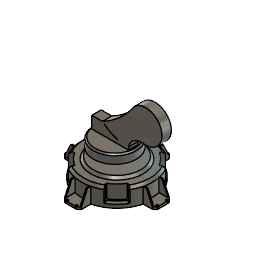
Robotic_Arm (Autodesk Fusion 360 design; units mm, degrees)
part number: 2026-03-02-22-55-42-666
part number: 2026-03-02-23-27-00-819
part number: 2026-03-03-10-06-11-483
part number: 2026-03-03-11-15-49-242
Autodesk Fusion 360 part; units mm, degrees
note: some values were not read from the file. Chosen so that the rebuilt part matches the saved one: which face or edge a step refers to; that a step has no effect. Set by a fixed rule: which sketch regions a step uses.
sketch "Sketch1" plane through (0, 0, 0) normal (0, 1, 0) x (1, 0, 0) in component "Base of thr Arm"
  circle A0 centre (0, 0) radius 150
  dimension "d1" = 300
  constraint coincident A0.centre origin
  measures "d1" diameter of A0
extrude "Extrude1" add sketch "Sketch1" along normal blind 75 makes body 1 in component "Base of thr Arm"
chamfer "Chamfer1" distance 10 angle 45 1 edges at (-139.8491, 75, 54.2423) on bodies 1 in component "Base of thr Arm"
sketch "Sketch1 (2)" plane through (0, 0, 0) normal (0, 1, 0) x (1, 0, 0)
  line L0 (-195.7386, 0) -> (-195.7386, 35.5)
  line L1 (-195.7386, 0) -> (-195.7386, -35.5)
  line L2 (-195.7386, 35.5) -> (-145.7386, 35.5)
  line L3 (-195.7386, -35.5) -> (-145.7386, -35.5)
  circle A0 centre (0, 0) radius 150
  dimension "d23" = 35.5
  dimension "d24" = 35.5
  dimension "d25" = 50
  dimension "d26" = 50
  constraint vertical L0
  constraint vertical L1
  constraint perpendicular L0 L2
  constraint perpendicular L1 L3
  constraint coincident L2.end A0
  constraint coincident L3.end A0
  measures "d23" distance of L0.start L0.end
  measures "d24" distance of L0.start L1.end
  measures "d25" distance of L0.end L2.end
  measures "d26" distance of L1.end L3.end
extrude "Extrude1'" add sketch "Sketch1 (2)" along normal blind 10 separate body contours L0 L1 L2 L3 A0 makes body 2 in component "Scerw holder"
sketch "Sketch1 (3)" plane through (0, 0, 35.5) normal (0, 0, 1) x (1, 0, 0) in component "Scerw holder"
  line L0 (-195.7386, 0) -> (-145.7386, 0)
  line L1 (-145.7386, 0) -> (-145.7386, 10)
  line L2 (-145.7386, 10) -> (-195.7386, 10)
  line L3 (-195.7386, 10) -> (-195.7386, 0)
  line L4 (-145.7386, 10) -> (-145.7386, 65)
  line L5 (-145.7386, 65) -> (-160, 65)
  line L6 (-160, 65) -> (-185, 10)
  line L7 (-145.7386, 10) -> (-185, 10)
  constraint coincident L1.end L2.start
  constraint perpendicular L2 L4
  constraint perpendicular L4 L5
  constraint coincident L2 L6.end
extrude "Extrude3" add sketch "Sketch1 (3)" against normal blind 5 contours L2 L4 L5 L6 L7 bodies 2 in component "Scerw holder"
chamfer "Chamfer2" distance 10.5 angle 45 2 edges at (-195.7386, 5, -35.5) (-195.7386, 5, 35.5) on bodies 2 in component "Scerw holder"
sketch "Sketch2" plane through (0, 10, 0) normal (0, 1, 0) x (-1, 0, 0) in component "Scerw holder"
  line L0 (195.7386, 25) -> (185.2386, 35.5)
  line L1 (185.2386, 35.5) -> (185, 35.5)
  line L2 (185, 35.5) -> (185, 30.5)
  line L3 (185, 30.5) -> (146.8664, 30.5)
  arc A0 (145.7386, -35.5) -> (146.8664, 30.5) centre (0, 0) ccw
  line L4 (145.7386, -35.5) -> (185.2386, -35.5)
  line L5 (185.2386, -35.5) -> (195.7386, -25)
  line L6 (195.7386, -25) -> (195.7386, 25)
  line L7 (194, 22.3094) -> (190, 24.6188)
  line L8 (190, 24.6188) -> (186, 22.3094)
  line L9 (186, 22.3094) -> (186, 17.6906)
  line L10 (186, 17.6906) -> (190, 15.3812)
  line L11 (190, 15.3812) -> (194, 17.6906)
  line L12 (194, 17.6906) -> (194, 22.3094)
  point P0 (190, 20)
extrude "Extrude4" cut sketch "Sketch2" against normal blind 10 contours L7 L8 L9 L10 L11 L12 bodies 2 in component "Scerw holder"
mirror "Mirror2" about plane through (0, 0, 0) normal (0, 0, 1) of "Extrude3", "Extrude4" in component "Scerw holder"
pattern_circular "C-Pattern1" count 4 over 360 about axis through (0, 1.75, 0) along (0, 1, 0) of bodies 2 makes body 3 at (0, 0, 174) makes body 4 at (174, 0, 0) makes body 5 at (0, 0, -174) in component "Scerw holder"
sketch "Sketch5" plane through (0, 75, 0) normal (0, 1, 0) x (-1, 0, 0) in component "Base of thr Arm"
  circle A0 centre (0, 0) radius 140
  line L0 (0, 0) -> (170, 0)
  line L1 (0, 0) -> (0, 150)
  line L2 (0, 0) -> (174.0838, 100.5073)
  line L3 (0, 0) -> (105.4587, 182.6598)
  circle A1 centre (0, 0) radius 130
  circle A2 centre (0, 0) radius 150
  dimension "d47" = 30
  dimension "d48" = 30
  dimension "d49" = 260
  dimension "d50" = 300
  constraint coincident A0.centre L0.start
  constraint horizontal L0
  constraint perpendicular L0 L1
  measures "d47" angle of L0 L2
  measures "d48" angle of L1 L3
  measures "d49" diameter of A1
  measures "d50" diameter of A2
extrude "Extrude6" cut sketch "Sketch5" against normal blind 60 contours A0 L2 L3 A1 | A0 L2 L3 A2 bodies 1 in component "Base of thr Arm"
fillet "Fillet1" radius 3 5 edges at (-112.5833, 45, 65) (-65, 45, 112.5833) (-91.9239, 15, 91.9239) (-121.2436, 15, 70) (-70, 15, 121.2436) on bodies 1 in component "Base of thr Arm"
pattern_circular "C-Pattern1'" count 4 over 360 about axis through (0, 1.75, 0) along (0, 1, 0) of 11 faces at (-105.3564, 37, 76.1579) (-112.4433, 37, 66.3355) (-112.3586, 17.6084, 66.4028) (-123.6174, 15.0142, 74.498) (-120.0379, 15, 79.7213) (-76.2075, 17.2927, 105.4249) (-66.1107, 17.6084, 113.5001) (-66.2488, 37, 114.641) (-69.3221, 52.6667, 120.0693) (-73.7477, 15.2347, 124.0613) (-120.0693, 52.6667, 69.3221) on bodies 1 in component "Base of thr Arm"
sketch "Sketch6" plane through (0, 75, 0) normal (0, 1, 0) x (-1, 0, 0) in component "Base of thr Arm"
  line L0 (115.1521, -66.4831) -> (121.2436, -70)
  arc A0 (121.2436, -70) -> (121.2436, 70) centre (0, 0) ccw
  line L1 (121.2436, 70) -> (115.1521, 66.4831)
  arc A1 (111.0885, 67.5229) -> (115.1521, 66.4831) centre (113.6521, 69.0812) ccw
  arc A2 (111.0885, 67.5229) -> (67.5229, 111.0885) centre (0, 0) ccw
  arc A3 (66.4831, 115.1521) -> (67.5229, 111.0885) centre (69.0812, 113.6521) ccw
  line L2 (66.4831, 115.1521) -> (70, 121.2436)
  arc A4 (70, 121.2436) -> (-70, 121.2436) centre (0, 0) ccw
  line L3 (-70, 121.2436) -> (-66.4831, 115.1521)
  arc A5 (-67.5229, 111.0885) -> (-66.4831, 115.1521) centre (-69.0812, 113.6521) ccw
  arc A6 (-67.5229, 111.0885) -> (-111.0885, 67.5229) centre (0, 0) ccw
  arc A7 (-115.1521, 66.4831) -> (-111.0885, 67.5229) centre (-113.6521, 69.0812) ccw
  line L4 (-115.1521, 66.4831) -> (-121.2436, 70)
  arc A8 (-121.2436, 70) -> (-121.2436, -70) centre (0, 0) ccw
  line L5 (-121.2436, -70) -> (-115.1521, -66.4831)
  arc A9 (-111.0885, -67.5229) -> (-115.1521, -66.4831) centre (-113.6521, -69.0812) ccw
  arc A10 (-111.0885, -67.5229) -> (-67.5229, -111.0885) centre (0, 0) ccw
  arc A11 (-66.4831, -115.1521) -> (-67.5229, -111.0885) centre (-69.0812, -113.6521) ccw
  line L6 (-66.4831, -115.1521) -> (-70, -121.2436)
  arc A12 (-70, -121.2436) -> (70, -121.2436) centre (0, 0) ccw
  line L7 (70, -121.2436) -> (66.4831, -115.1521)
  arc A13 (67.5229, -111.0885) -> (66.4831, -115.1521) centre (69.0812, -113.6521) ccw
  arc A14 (67.5229, -111.0885) -> (111.0885, -67.5229) centre (0, 0) ccw
  arc A15 (115.1521, -66.4831) -> (111.0885, -67.5229) centre (113.6521, -69.0812) ccw
  circle A16 centre (0, 0) radius 110
  dimension "d57" = 220
  constraint concentric A0 A16
  measures "d57" diameter of A16
extrude "Extrude7" add sketch "Sketch6" along normal blind 10 draft -45 contours A16 bodies 1 in component "Base of thr Arm"
sketch "Sketch7" plane through (0, 85, 0) normal (0, 1, 0) x (-1, 0, 0) in component "Base of thr Arm"
  circle A0 centre (0, 0) radius 100
  circle A1 centre (0, 0) radius 15
  dimension "d60" = 30
  constraint coincident A0.centre A1.centre
  measures "d60" diameter of A1
extrude "Extrude8" add sketch "Sketch7" along normal blind 20 contours A1 bodies 1 in component "Base of thr Arm"
sketch "Sketch1 (4)" plane through (0, 0, 0) normal (0, 1, 0) x (1, 0, 0) in component "Arm Jaw"
  circle A0 centre (0, 0) radius 90
  dimension "d63" = 180
  constraint coincident A0.centre origin
  measures "d63" diameter of A0
extrude "Extrude1''" add sketch "Sketch1 (4)" along normal blind 37 separate body makes body 6 in component "Arm Jaw"
chamfer "Chamfer1'" distance 6 angle 45 1 edges at (-83.9095, 37, 32.5454) on bodies 6 in component "Arm Jaw"
sketch "Sketch2 (2)" plane through (0, 37, 0) normal (0, 1, 0) x (-1, 0, 0) in component "Arm Jaw"
  circle A0 centre (0, 0) radius 84
  line L0 (77.5, 20) -> (-77.5, 20)
  line L1 (-77.5, 20) -> (-77.5, -20)
  line L2 (-77.5, -20) -> (77.5, -20)
  line L3 (77.5, -20) -> (77.5, 20)
  line L4 (77.5, 20) -> (-77.5, -20) construction
  line L5 (-77.5, 20) -> (77.5, -20) construction
  dimension "d67" = 155
  dimension "d68" = 40
  constraint horizontal L0
  constraint perpendicular L0 L1
  constraint parallel L0 L2
  constraint parallel L1 L3
  constraint coincident L4 A0.centre
  constraint coincident L5 A0.centre
  constraint coincident A0.centre origin
  measures "d67" distance of L1.end L2.end
  measures "d68" distance of L0.end L1.end
extrude "Extrude2" add sketch "Sketch2 (2)" along normal blind 50 contours L0 L1 L2 L3 bodies 6 in component "Arm Jaw"
sketch "Sketch3" plane through (0, 0, -20) normal (0, 0, -1) x (-1, 0, 0) in component "Arm Jaw"
  line L0 (-77.5, 37) -> (77.5, 37)
  line L1 (77.5, 37) -> (77.5, 87)
  line L2 (77.5, 87) -> (-77.5, 87)
  line L3 (-77.5, 87) -> (-77.5, 37)
  line L4 (-77.5, 87) -> (5.9265, 87)
  line L5 (-77.5, 87) -> (32.5, 87)
  line L6 (-77.5, 87) -> (-77.5, 48)
  arc A0 (-77.5, 48) -> (32.5, 87) centre (-70.2732, 202.2449) ccw
  dimension "d71" = 110
  dimension "d72" = 39
  constraint coincident L2.end L3.start
  constraint coincident L2 L4.end
  constraint perpendicular L3 L5
  constraint perpendicular L5 L6
  measures "d71" distance of L2.end L5.end
  measures "d72" distance of L2.end L6.end
extrude "Extrude3'" cut sketch "Sketch3" against normal blind 80 contours L2 L3 L4 L5 L6 A0 bodies 6 in component "Arm Jaw"
sketch "Sketch4" plane through (0, 0, 0) normal (0, 0, 1) x (1, 0, 0) in component "Arm Jaw"
  line L0 (0, 0) -> (150, 0)
  line L1 (150, 0) -> (150, 160)
  circle A0 centre (150, 160) radius 68.5
  arc A1 (139.9423, 92.2424) -> (77.3691, 47.5292) centre (131.8134, 37.4782) ccw
  arc A2 (-32.5378, 86.9467) -> (99.6249, 206.4177) centre (-205.8032, 411.4553) ccw
  arc A3 (-32.5378, 86.9467) -> (77.3691, 47.5292) centre (72.3379, 206.4349) ccw
  dimension "d75" = 160
  dimension "d76" = 137
  constraint coincident L0.start origin
  constraint horizontal L0
  constraint perpendicular L0 L1
  constraint coincident L1.end A0.centre
  constraint tangent A0 A1
  constraint coincident A0 A1.start
  constraint coincident A0 A2.end
  constraint tangent A0 A3
  measures "d75" distance of L0.end L1.end
  measures "d76" diameter of A0
extrude "Extrude4'" add sketch "Sketch4" along normal mid plane 40 contours A0 A2 | A0 A1 A2 A3 picked at (167.4331, 144.9511) bodies 6 in component "Arm Jaw"
sketch "Sketch2 (3)" plane through (0, 0, 35.5) normal (0, 0, 1) x (1, 0, 0)
  line L0 (-185.2386, 0) -> (-145.7386, 0)
  line L1 (-145.7386, 0) -> (-145.7386, 10)
  line L2 (-185, 10) -> (-185.2386, 10)
  line L3 (-145.7386, 10) -> (-145.7386, 65)
  line L4 (-145.7386, 65) -> (-160, 65)
  line L5 (-160, 65) -> (-185, 10)
  line L6 (-185, 10) -> (-145.7386, 10)
  line L7 (-185.2386, 10) -> (-185.2386, 0)
  line L8 (-145.7386, 10) -> (-145.7386, 65)
  line L9 (-145.7386, 65) -> (-160, 65)
  line L10 (-160, 65) -> (-185, 10)
  constraint coincident L1.end L3.start
  constraint perpendicular L2 L3
  constraint perpendicular L1 L4
  constraint coincident L2 L5.end
extrude "Extrude5" add sketch "Sketch2 (3)" against normal blind 5 contours L3 L4 L5 L6 L8 L9 L10 bodies 1 in component "Base of thr Arm"
chamfer "Chamfer1''" [no effect] in component "Scerw holder"
sketch "Sketch3 (2)" plane through (0, 10, 0) normal (0, 1, 0) x (-1, 0, 0)
  line L0 (195.7386, -25) -> (195.7386, 25)
  line L1 (185.2386, 35.5) -> (185, 35.5)
  arc A0 (146.8664, -30.5) -> (146.8664, 30.5) centre (0, 0) ccw
  line L2 (185, -35.5) -> (185.2386, -35.5)
  line L3 (194, 22.3094) -> (190, 24.6188)
  line L4 (190, 24.6188) -> (186, 22.3094)
  line L5 (186, 22.3094) -> (186, 17.6906)
  line L6 (186, 17.6906) -> (190, 15.3812)
  line L7 (190, 15.3812) -> (194, 17.6906)
  line L8 (194, 17.6906) -> (194, 22.3094)
  line L9 (194, -22.3094) -> (190, -24.6188)
  line L10 (190, -24.6188) -> (186, -22.3094)
  line L11 (186, -22.3094) -> (186, -17.6906)
  line L12 (186, -17.6906) -> (190, -15.3812)
  line L13 (190, -15.3812) -> (194, -17.6906)
  line L14 (194, -17.6906) -> (194, -22.3094)
  line L15 (146.8664, -30.5) -> (185, -30.5)
  line L16 (185, -30.5) -> (185, -35.5)
  line L17 (185.2386, -35.5) -> (195.7386, -25)
  line L18 (195.7386, 25) -> (185.2386, 35.5)
  line L19 (185, 35.5) -> (185, 30.5)
  line L20 (185, 30.5) -> (146.8664, 30.5)
  line L21 (190, 24.6188) -> (194, 22.3094)
  line L22 (194, 22.3094) -> (194, 17.6906)
  line L23 (194, 17.6906) -> (190, 15.3812)
  line L24 (190, 15.3812) -> (186, 17.6906)
  line L25 (186, 17.6906) -> (186, 22.3094)
  line L26 (186, 22.3094) -> (190, 24.6188)
  point P0 (190, 20)
extrude "Extrude2'" cut sketch "Sketch3 (2)" against normal blind 17 contours L3 L4 L5 L6 L7 L8 L21 L22 L23 L24 L25 L26 bodies 2 in component "Scerw holder"
mirror "Mirror2'" about plane through (0, 0, 0) normal (0, 0, 1) of "Extrude5" in component "Base of thr Arm"
sketch "Sketch4 (2)" plane through (-26.7868, -149.2699, 20) normal (0, 0, 1) x (1, 0, 0)
  arc A0 (166.7292, 241.5123) -> (104.2446, 197.2679) centre (158.6002, 186.7481) ccw
  arc A1 (166.7292, 241.5123) -> (126.4118, 355.6876) centre (176.7868, 309.2699) ccw
  arc A2 (-5.6899, 236.2492) -> (126.4118, 355.6876) centre (-179.0163, 560.7252) ccw
  arc A3 (-5.7132, 236.2699) -> (-5.6899, 236.2492) centre (97.0582, 351.5128) ccw
  line L0 (-5.7132, 236.2699) -> (-50.7132, 236.2699)
  line L1 (-50.7132, 236.2699) -> (-50.7132, 186.2699)
  line L2 (-50.7132, 186.2699) -> (104.2868, 186.2699)
  line L3 (104.2868, 186.2699) -> (104.2868, 197.2699)
  arc A4 (104.2446, 197.2679) -> (104.2868, 197.2699) centre (97.06, 351.515) ccw
sketch "Sketch5 (2)" plane through (0, 0, -20) normal (0, 0, -1) x (-1, 0, 0) in component "Arm Jaw"
  arc A0 (-77.5, 48) -> (-77.4578, 47.998) centre (-70.2732, 202.2449) ccw
  line L0 (-77.5, 48) -> (-77.5, 37)
  line L1 (-77.5, 37) -> (77.5, 37)
  line L2 (77.5, 37) -> (77.5, 87)
  line L3 (77.5, 87) -> (32.5, 87)
  arc A1 (32.4768, 86.9793) -> (32.5, 87) centre (-70.2732, 202.2449) ccw
  arc A2 (-99.6249, 206.4177) -> (32.4768, 86.9793) centre (205.8032, 411.4553) ccw
  arc A3 (-99.6249, 206.4177) -> (-139.9423, 92.2424) centre (-150, 160) ccw
  arc A4 (-77.4578, 47.998) -> (-139.9423, 92.2424) centre (-131.8134, 37.4782) ccw
  arc A5 (-32.4241, 52.5413) -> (25.3825, 81.0273) centre (-72.3379, 206.4349) ccw
  arc A6 (-32.4241, 52.5413) -> (25.3825, 81.0273) centre (-70.2732, 202.2449) ccw
  circle A7 centre (-150, 160) radius 55
  dimension "d79" = 110
  constraint concentric A3 A7
  measures "d79" diameter of A7
extrude "Extrude5'" add sketch "Sketch5 (2)" along normal blind 20 draft -40 contours A7 bodies 6 in component "Arm Jaw"
sketch "Sketch6 (2)" plane through (0, 0, -40) normal (0, 0, -1) x (-1, 0, 0) in component "Arm Jaw"
  circle A0 centre (-150, 160) radius 38.218
  line L0 (-150, 160) -> (-150, 224)
  arc A1 (-158.9698, 214.2636) -> (-150, 206) centre (-150, 215) ccw
  circle A2 centre (-150, 160) radius 55
  arc A3 (-150, 206) -> (-141.0302, 214.2636) centre (-150, 215) ccw
  dimension "d82" = 9
  dimension "d83" = 9
  constraint coincident A0.centre L0.start
  constraint vertical L0
  constraint coincident L0 A1.end
  constraint coincident L0 A1.centre
  constraint coincident A1.start A2
  constraint coincident A1.centre A2
  constraint coincident A2 A3.end
  constraint coincident A1.centre A3.centre
  measures "d82" distance of L0.end A1.centre
  measures "d83" distance of A1.end A1.centre
extrude "Extrude6'" cut sketch "Sketch6 (2)" against normal blind 20 contours L0 A1 A2 | L0 A2 A3 bodies 6 in component "Arm Jaw"
sketch "Sketch7 (2)" plane through (0, 0, -20) normal (0, 0, -1) x (-1, 0, 0) in component "Arm Jaw"
  arc A0 (-158.9698, 214.2636) -> (-141.0302, 214.2636) centre (-150, 160) ccw
  arc A1 (-158.9698, 214.2636) -> (-141.0302, 214.2636) centre (-150, 215) ccw
  arc A2 (-77.5, 48) -> (-77.4578, 47.998) centre (-70.2732, 202.2449) ccw
  line L0 (-77.5, 48) -> (-77.5, 37)
  line L1 (-77.5, 37) -> (77.5, 37)
  line L2 (77.5, 37) -> (77.5, 87)
  line L3 (77.5, 87) -> (32.5, 87)
  arc A3 (32.4768, 86.9793) -> (32.5, 87) centre (-70.2732, 202.2449) ccw
  arc A4 (-99.6249, 206.4177) -> (32.4768, 86.9793) centre (205.8032, 411.4553) ccw
  arc A5 (-99.6249, 206.4177) -> (-139.9423, 92.2424) centre (-150, 160) ccw
  arc A6 (-77.4578, 47.998) -> (-139.9423, 92.2424) centre (-131.8134, 37.4782) ccw
  arc A7 (-32.4241, 52.5413) -> (25.3825, 81.0273) centre (-72.3379, 206.4349) ccw
  arc A8 (-32.4241, 52.5413) -> (25.3825, 81.0273) centre (-70.2732, 202.2449) ccw
  circle A9 centre (-150, 215) radius 4.1231
  line L4 (-154.1231, 212.6195) -> (-150, 210.239)
  line L5 (-150, 210.239) -> (-145.8769, 212.6195)
  line L6 (-145.8769, 212.6195) -> (-145.8769, 217.3805)
  line L7 (-145.8769, 217.3805) -> (-150, 219.761)
  line L8 (-150, 219.761) -> (-154.1231, 217.3805)
  line L9 (-154.1231, 217.3805) -> (-154.1231, 212.6195)
  circle A10 centre (-150, 215) radius 2.5
  point P0 (-150, 215)
  dimension "d86" = 5
  constraint concentric A1 A9
  constraint coincident P0 A1.centre
  constraint concentric A9 A10
  measures "d86" diameter of A10
extrude "Extrude7'" add sketch "Sketch7 (2)" along normal blind 1 contours A9 | A9 L5 L6 | A9 L6 L7 | A9 L7 L8 | A9 L4 L5 | A9 L8 L9 | A9 L4 L9 bodies 6 in component "Arm Jaw"
pattern_circular "C-Pattern1''" count 8 over 360 about axis through (150, 160, -40) along (0, 0, 1) of "Extrude6'", "Extrude7'" in component "Arm Jaw"
component "Base of thr Arm" placed x (1, 0, 0) y (0, 1, 0) z (0, 0, 1) at (0, 0, 0)
component "Arm Jaw" placed x (1, 0, 0) y (0, 1, 0) z (0, 0, 1) at (0, 0, 0)
component "Scerw holder" placed x (1, 0, 0) y (0, 1, 0) z (0, 0, 1) at (0, 0, 0) in component "Base of thr Arm"
